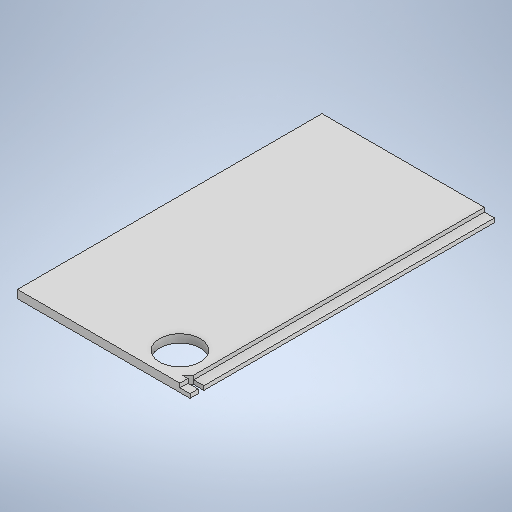
# Autodesk Inventor part: backWall
Saved by Autodesk Inventor 2026.1 (Build 301233000, 233)
## iProperties
Created: 2026-08-16
Part Number: backWall
Material: Generic
Document SubType Name: Modeling
Designer: rowan
Density: 1 g/cm^3
Appearance: Default
Author: rowan
Autodesk Inventor part; units mm, degrees
ref_plane "YZ Plane" through (0, 0, 0) normal (1, 0, 0) x (0, 1, 0)
ref_plane "XZ Plane" through (0, 0, 0) normal (0, 1, 0) x (-1, 0, 0)
ref_plane "XY Plane" through (0, 0, 0) normal (0, 0, 1) x (1, 0, 0)
sketch "Sketch1" plane through (0, 0, 0) normal (0, 1, 0) x (-1, 0, 0)
  line L0 (0, 0) -> (80, 0)
  line L1 (80, 0) -> (80, -150)
  line L2 (80, -150) -> (0, -150)
  line L3 (0, -150) -> (0, 0)
  line L4 (0, 0) -> (-5, 0)
  line L5 (-5, 0) -> (-5, -150)
  line L6 (-5, -150) -> (0, -150)
  line L7 (0, -150) -> (0, 0)
  line L8 (0, -6.8284) -> (2.8284, -4)
  circle A0 centre (14, -14) radius 10
  line L9 (2.8284, -4) -> (0, -4)
  line L10 (0, -6.8284) -> (-5, -6.8284)
  line L11 (0, -4) -> (-5, -4)
  dimension "d0" = 150
  dimension "d1" = 80
  dimension "d2" = 5
  dimension "d3" = 4
  dimension "d4" = 45
  dimension "d5" = 20
  dimension "d6" = 4
  dimension "d7" = 14
  dimension "d8" = 14
  constraints: 24 end point, 5 perpendicular, 4 parallel, 4 point on line, 2 horizontal, 1 centre point
  measures "d0" distance of L2.end L0.start
  measures "d1" distance of L0.start L0.end
  measures "d2" distance of L5.end L6.end
  measures "d3" distance of L8.start L8.end
  measures "d4" angle of L3 L8
  measures "d5" diameter of A0
  measures "d6" distance from line of L0 L8.end
  measures "d7" distance from line of L0 A0.centre
  measures "d8" distance from line of L3 A0.centre
extrude "Extrusion1" add sketch "Sketch1" along normal blind 4 contours L0 L1 L2 L3 L8 L9 | L9 L8 L3
extrude "Extrusion2" cut sketch "Sketch1" along normal blind 4 contours L9 L8 L3
extrude "Extrusion3" add sketch "Sketch1" along normal blind 2 contours L3 L11 L5 L4 | L3 L10 L5 L11 | L3 L6 L5 L10
extrude "Extrusion4" cut sketch "Sketch1" along normal blind 2 contours L3 L10 L5 L11
body "Solid1"
